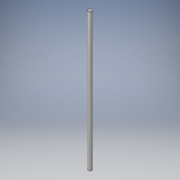
# Autodesk Inventor part: 8mm smooth rod
Saved by Autodesk Inventor 2016 (Build 200138000, 138)
## iProperties
Created: 2017-05-17
Part Number: 8mm smooth rod
Material: Generic
Document SubType Name: Modeling
Designer: 31745
Density: 1 g/cm^3
Appearance: Default
Author: 31745
Autodesk Inventor part; units mm, degrees
ref_plane "YZ Plane" through (0, 0, 0) normal (1, 0, 0) x (0, 1, 0)
ref_plane "XZ Plane" through (0, 0, 0) normal (0, 1, 0) x (-1, 0, 0)
ref_plane "XY Plane" through (0, 0, 0) normal (0, 0, 1) x (1, 0, 0)
sketch "Sketch1" plane through (0, 0, 0) normal (0, 1, 0) x (-1, 0, 0)
  circle A0 centre (0, 0) radius 4
  dimension "d0" = 8
  constraints: 1 centre point, 1 coincident
  measures "d0" diameter of A0
extrude "Extrusion1" add sketch "Sketch1" along normal blind 279.4
chamfer "Chamfer1" distance 0.635 angle 45 2 edges at (4, 279.4, 0) (4, 0, 0)
body "Solid1"
